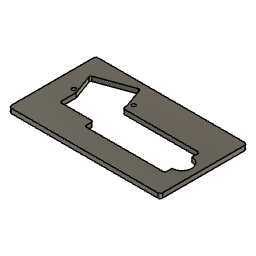
bevestigingsplankje achtervleugel v5 (Autodesk Fusion 360 design; units mm, degrees)
Autodesk Fusion 360 part; units mm, degrees
sketch "Sketch1" plane through (0, 0, 0) normal (0, 0, 1) x (1, 0, 0)
  line L0 (72.4034, 27.9167) -> (178.4034, 27.9167)
  line L1 (72.4034, 27.9167) -> (72.4034, 39.1667)
  line L2 (72.4034, 39.1667) -> (28.4034, 39.1667)
  line L3 (28.4034, 39.1667) -> (28.4034, 60.6444)
  line L4 (51.7694, 73.8535) -> (80.618, 84.3536) construction
  line L5 (51.7694, 73.8535) -> (87.8768, 73.8535) construction
  line L6 (80.618, 84.3536) -> (22.8269, 63.3193) construction
  line L7 (80.618, 84.3536) -> (137.5254, 84.3536) construction
  line L8 (178.4034, 73.4926) -> (77.2668, 73.4926)
  line L9 (72.4034, 39.1667) -> (72.4034, 27.9167)
  arc A0 (178.4034, 37.4167) -> (178.4034, 63.4167) centre (178.4034, 50.4167) ccw
  line L10 (178.4034, 27.9167) -> (178.4034, 37.4167)
  line L11 (178.4034, 63.4167) -> (178.4034, 73.4926)
  line L12 (0, 0) -> (200, 0)
  line L13 (200, 0) -> (200, 115)
  line L14 (200, 115) -> (0, 115)
  line L15 (0, 115) -> (0, 0)
  circle A1 centre (80.618, 84.3536) radius 2.5
  circle A2 centre (22.8269, 63.3193) radius 2.5
  line L16 (178.4034, 73.4926) -> (178.4034, 27.9167) construction
  line L17 (178.4034, 50.4167) -> (28.4034, 50.4167)
  line L18 (75.7554, 82.5838) -> (66.8629, 107.0158)
  line L19 (75.7554, 82.5838) -> (66.8629, 107.0158)
  line L20 (66.8629, 107.0158) -> (17.9989, 89.2307)
  line L21 (17.9989, 89.2307) -> (26.8914, 64.7987)
  line L22 (75.7554, 82.5838) -> (75.7337, 82.5692)
  arc A3 (77.2668, 73.4926) -> (75.7316, 82.5751) centre (51.7694, 73.8535) ccw
  line L23 (26.8914, 64.7987) -> (28.4034, 60.6444)
  dimension "d3" = 106
  dimension "d5" = 26
  dimension "d8" = 11.25
  dimension "d9" = 44
  dimension "d11" = 30.7
  dimension "d12" = 20
  dimension "d14" = 61.5
  dimension "d15" = 200
  dimension "d16" = 115
  dimension "d17" = 5
  dimension "d18" = 5
  dimension "d27" = 26
  dimension "d28" = 26
  dimension "d29" = 52
  constraint horizontal L0
  constraint vertical L10
  constraint horizontal L8
  constraint perpendicular L0 L1
  constraint horizontal L2
  constraint vertical L3
  constraint horizontal L5
  constraint coincident L4.start L5.start
  constraint horizontal L7
  constraint coincident A0.end L10
  constraint collinear L10 L11
  constraint coincident A0.centre L10
  constraint horizontal L12
  constraint vertical L13
  constraint horizontal L14
  constraint vertical L15
  constraint coincident L4.end L6.start
  constraint coincident L6.end A2.centre
  constraint coincident A0.centre L17.start
  constraint coincident L3 L17.end
  constraint perpendicular L3 L17
  constraint coincident L4 L18.start
  constraint perpendicular L6 L18
  constraint perpendicular L19 L20
  constraint coincident L6 L21.end
  constraint perpendicular L6 L21
  constraint coincident L22.end A3
  constraint coincident L4 A3.end
  constraint perpendicular L6 L23
  constraint coincident L12.start L15.end
  measures "d3" distance of L0.start L0.end
  measures "d5" diameter of A0
  measures "d8" distance of L0.start L1.end
  measures "d9" distance of L1.end L2.end
  measures "d11" distance of L4.start L4.end
  measures "d12" angle of L4 L5
  measures "d14" distance of L4.end L6.end
  measures "d15" distance of L12.start L12.end
  measures "d16" distance of L12.start L14.end
  measures "d17" diameter of A1
  measures "d18" diameter of A2
  measures "d27" distance of L18.start L18.end
  measures "d28" distance of L18.end L18.start
  measures "d29" distance of L18.end L20.end
extrude "Extrude3" add sketch "Sketch1" along normal blind 6
fillet "Fillet3" radius 3 1 edges at (200, 0, 3)
fillet "Fillet4" radius 3 3 edges at (0, 0, 3) (0, 115, 3) (200, 115, 3)
fillet "Fillet5" radius 2 7 edges at (17.9989, 89.2307, 3) (66.8629, 107.0158, 3) (77.2668, 73.4926, 3) (28.4034, 39.1667, 3) (72.4034, 27.9167, 3) (178.4034, 27.9167, 3) (178.4034, 73.4926, 3)
fillet "Fillet6" radius 2 1 edges at (72.4034, 39.1667, 3)
